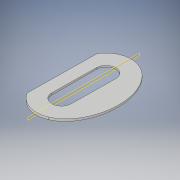
# Autodesk Inventor part: SPD_MTB_cleat_new
Saved by Autodesk Inventor 2019 (Build 230136000, 136)
## iProperties
Created: 2019-05-09
Part Number: SPD_MTB_cleat_new
Material: Generic
Document SubType Name: Modeling
Designer: assman
Density: 1 g/cm^3
Appearance: Default
Author: assman
Autodesk Inventor part; units mm, degrees
ref_plane "YZ Plane" through (0, 0, 0) normal (1, 0, 0) x (0, 1, 0)
ref_plane "XZ Plane" through (0, 0, 0) normal (0, 1, 0) x (-1, 0, 0)
ref_plane "XY Plane" through (0, 0, 0) normal (0, 0, 1) x (1, 0, 0)
sketch "Sketch1" plane through (0, 0, 0) normal (0, 1, 0) x (-1, 0, 0)
  line L0 (0, 0) -> (0, -34.15) construction
  arc A0 (6.6649, -3.975) -> (-7.575, -7.575) centre (0, -7.575) ccw construction
  arc A1 (-7.575, -26.575) -> (6.6649, -30.175) centre (0, -26.575) ccw construction
  line L1 (4.075, -7.575) -> (4.075, -26.575) construction
  arc A2 (-4.075, -26.575) -> (4.075, -26.575) centre (0, -26.575) ccw construction
  line L2 (-4.075, -26.575) -> (-4.075, -7.575) construction
  arc A3 (4.075, -7.575) -> (-4.075, -7.575) centre (0, -7.575) ccw construction
  line L3 (9.1649, -3.975) -> (9.1649, -30.175) construction
  line L4 (9.1649, -3.975) -> (6.6649, -3.975) construction
  line L5 (9.1649, -30.175) -> (6.6649, -30.175) construction
  line L6 (-10.575, -14.075) -> (-10.575, -20.075) construction
  line L7 (0, -17.075) -> (-19.3792, -17.075) construction
  line L8 (-4.075, -20.075) -> (-4.075, -24.075) construction
  line L9 (-10.575, -20.075) -> (-7.575, -21.8932) construction
  line L10 (-10.575, -14.075) -> (-7.575, -12.2568) construction
  line L11 (-7.575, -7.575) -> (-7.575, -12.2568) construction
  line L12 (-7.575, -21.8932) -> (-7.575, -26.575) construction
  line L13 (-10.575, -17.075) -> (-16.875, -17.075) construction
  line L14 (-10.575, -14.075) -> (-14.875, -14.075) construction
  line L15 (-16.875, -16.075) -> (-16.875, -18.075) construction
  line L16 (-14.875, -20.075) -> (-10.575, -20.075) construction
  arc A4 (-14.875, -14.075) -> (-16.875, -16.075) centre (-14.875, -16.075) ccw construction
  arc A5 (-16.875, -18.075) -> (-14.875, -20.075) centre (-14.875, -18.075) ccw construction
  line L17 (-6.7059, -17.075) -> (-6.7059, -23.075) construction
  line L18 (-6.7059, -17.075) -> (-6.7059, -11.075) construction
  line L19 (-7.575, -11.075) -> (-14.875, -11.075) construction
  line L20 (-16.875, -13.075) -> (-16.875, -21.075) construction
  line L21 (-14.875, -23.075) -> (-7.575, -23.075) construction
  arc A6 (-14.875, -11.075) -> (-16.875, -13.075) centre (-14.875, -13.075) ccw construction
  arc A7 (-16.875, -21.075) -> (-14.875, -23.075) centre (-14.875, -21.075) ccw construction
  line L22 (19.3047, -16.075) -> (19.3047, -18.075) construction
  line L23 (17.3047, -14.075) -> (13.3047, -14.075) construction
  line L24 (17.3047, -20.075) -> (13.3047, -20.075) construction
  line L25 (9.1649, -16.075) -> (9.1649, -22.575) construction
  line L26 (9.1649, -17.075) -> (9.1649, -11.575) construction
  line L27 (9.1649, -11.575) -> (13.3047, -14.075) construction
  line L28 (9.1649, -22.575) -> (13.3047, -20.075) construction
  arc A8 (19.3047, -16.075) -> (17.3047, -14.075) centre (17.3047, -16.075) ccw construction
  arc A9 (17.3047, -20.075) -> (19.3047, -18.075) centre (17.3047, -18.075) ccw construction
  line L29 (9.1649, -30.175) -> (9.1649, -26.175) construction
  line L30 (9.1649, -3.975) -> (9.1649, -7.975) construction
  line L31 (9.1649, -24.9114) -> (13.8618, -22.075) construction
  line L32 (13.8618, -22.075) -> (17.3047, -22.075) construction
  arc A10 (17.3047, -22.075) -> (21.3047, -18.075) centre (17.3047, -18.075) ccw construction
  line L33 (21.3047, -18.075) -> (21.3047, -16.075) construction
  arc A11 (21.3047, -16.075) -> (17.3047, -12.075) centre (17.3047, -16.075) ccw construction
  line L34 (17.3047, -12.075) -> (13.8618, -12.075) construction
  line L35 (13.8618, -12.075) -> (9.1649, -9.2386) construction
  point P0 (7.575, -17.075)
  point P1 (-4.075, -10.075)
  point P2 (19.3047, -14.075)
  point P3 (19.3047, -20.075)
  dimension "d0" = 34.15
  dimension "d1" = 15.15
  dimension "d5" = 6
  dimension "d7" = 4
  dimension "d8" = 2.5
  dimension "d9" = 3.5
  dimension "d10" = 8.15
  dimension "d12" = 2
  dimension "d14" = 6
  dimension "d15" = 6
  dimension "d16" = 2
  dimension "d18" = 6
  dimension "d19" = 6
  dimension "d20" = 5.5
  dimension "d21" = 5.5
  dimension "d23" = 4
  dimension "d24" = 4
  dimension "d25" = 2
  constraints: 72 end point, 26 point on circle, 16 tangent, 15 point on line, 12 centre point, 6 horizontal, 4 perpendicular, 3 vertical, 2 equal radius, 2 midpoint, 2 parallel, 1 symmetric about line, 14 other
  measures "d0" distance of L0.start L0.end
  measures "d1" diameter of A1
  measures "d5" distance of L6.start L6.end
  measures "d7" distance of L8.start L8.end
  measures "d8" distance of L5.start L5.end
  measures "d9" radial gap between concentric circles of A1 A2
  measures "d10" distance between parallel lines of L1 L2
  measures "d12" radius of A4
  measures "d14" distance of L17.start L17.end
  measures "d15" distance of L17.start L18.end
  measures "d16" radius of A6
  measures "d18" distance of point (19.305, -14.075) point (19.305, -20.075)
  measures "d19" distance of L23.end point (19.305, -14.075)
  measures "d20" distance of L26.start L25.end
  measures "d21" distance of L26.start L26.end
  measures "d23" distance of L5.start L29.end
  measures "d24" distance of L4.start L30.end
  measures "d25" radial gap between concentric circles of A9 A10
sketch "Sketch3" plane through (0, 0, 0) normal (0, 1, 0) x (-1, 0, 0)
  arc A0 (6.6649, -3.975) -> (-7.575, -7.575) centre (0, -7.575) ccw construction
  arc A1 (-7.575, -26.575) -> (6.6649, -30.175) centre (0, -26.575) ccw construction
  arc A2 (-4.075, -26.575) -> (4.075, -26.575) centre (0, -26.575) ccw projected
  line L0 (4.075, -7.575) -> (4.075, -26.575) projected
  arc A3 (4.075, -7.575) -> (-4.075, -7.575) centre (0, -7.575) ccw projected
  line L1 (-4.075, -26.575) -> (-4.075, -7.575) projected
  line L2 (9.1649, -3.975) -> (9.1649, -30.175) construction
  line L3 (-10.575, -14.075) -> (-10.575, -20.075) construction
  line L4 (-16.875, -16.075) -> (-16.875, -18.075) construction
  arc A4 (8.836, -1.765) -> (-4.3309, 2.0725) centre (0, -7.575) ccw
  arc A5 (-4.3309, -36.2225) -> (8.836, -32.385) centre (0, -26.575) ccw
  line L5 (9.1649, -2.8638) -> (9.1649, -31.2862)
  arc A6 (9.1649, -2.8638) -> (8.836, -1.765) centre (7.1649, -2.8638) ccw
  arc A7 (8.836, -32.385) -> (9.1649, -31.2862) centre (7.1649, -31.2862) ccw
  line L6 (-12.075, -10.8843) -> (-12.075, -24.6972)
  ellipse E0 centre (0, -17.075) end of major axis (0, -37.15) minor radius 14.4147 (-4.3309, 2.0725) -> (-4.3309, -36.2225) ccw
  point P0 (0, 0)
  point P1 (9.1649, -2.2991)
  point P2 (9.1649, -31.8509)
  dimension "d26" = 3
  dimension "d27" = 3
  dimension "d28" = 2
  dimension "d29" = 6.5
  dimension "d30" = 8
  constraints: 10 point on circle, 4 centre point, 4 end point, 4 point on line, 4 tangent, 1 equal radius, 1 vertical, 4 other
  measures "d26" radial gap between concentric circles of A0 A4
  measures "d27" radial gap between concentric circles of A1 A5
  measures "d28" radius of A6
  measures "d29" distance between parallel lines of L3 L1
  measures "d30" distance between parallel lines of L6 L1
extrude "Extrusion1" add sketch "Sketch3" along normal blind 1
ref_plane "Work Plane1" through (0, 1, 3) normal (1, 0, 0) x (0, 0, -1)
sketch "Sketch7" plane through (0, 1, 3) normal (1, 0, 0) x (0, 0, -1)
  line L0 (40.15, 0) -> (40.15, -1) projected
  line L1 (40.15, -1) -> (33.65, -1) projected
  line L2 (33.65, -1) -> (33.65, 0) projected
  line L3 (33.65, 0) -> (40.15, 0) projected
  line L4 (0, -1) -> (0, 0) projected
  line L5 (0, 0) -> (6.5, 0) projected
  line L6 (6.5, 0) -> (6.5, -1) projected
  line L7 (6.5, -1) -> (0, -1) projected
  line L8 (40.15, -1) -> (35.385, -1) construction
  line L9 (40.15, -1) -> (40.15, -0.5) construction
  line L10 (40.15, -1) -> (40.15, 0) construction
  line L11 (4.765, 0) -> (0, 0) construction
  line L12 (40.15, -0.5) -> (0, 0)
  line L13 (0, 0) -> (40.15, 0)
  line L14 (40.15, 0) -> (40.15, -0.5)
  point P0 (3, -1)
  point P1 (39.2225, -1)
  point P2 (0.9275, 0)
  constraints: 8 end point, 1 collinear, 1 horizontal, 1 midpoint
extrude "Extrusion2" cut sketch "Sketch7" along normal blind 20 and the other way blind 20 contours L0 L12 L2 L3 | L2 L12 L6 L13 | L6 L12 L5
body "Solid1"
